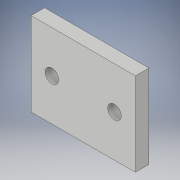
# Autodesk Inventor part: Bed Plate
Saved by Autodesk Inventor 2018 (Build 220112000, 112)
## iProperties
Created: 2017-04-14
Part Number: Bed Plate
Material: Generic
Document SubType Name: Modeling
Designer: Administrator
Density: 1 g/cm^3
Appearance: Default
Author: Administrator
Autodesk Inventor part; units mm, degrees
ref_plane "YZ Plane" through (0, 0, 0) normal (1, 0, 0) x (0, 1, 0)
ref_plane "XZ Plane" through (0, 0, 0) normal (0, 1, 0) x (-1, 0, 0)
ref_plane "XY Plane" through (0, 0, 0) normal (0, 0, 1) x (1, 0, 0)
sketch "Sketch1" plane through (0, 0, 0) normal (0, 0, 1) x (1, 0, 0)
  line L0 (-25, -20) -> (25, -20)
  line L1 (25, -20) -> (25, 20)
  line L2 (25, 20) -> (-25, 20)
  line L3 (-25, 20) -> (-25, -20)
  point P0 (0, 0)
  dimension "d0" = 50
  dimension "d1" = 40
  constraints: 8 end point, 2 parallel, 1 horizontal, 1 perpendicular
  measures "d0" distance of L2.end L1.end
  measures "d1" distance of L1.end L0.end
extrude "Extrusion1" add sketch "Sketch1" along normal blind 6.5
sketch "Sketch2" plane through (0, 0, 6.5) normal (0, 0, 1) x (1, 0, 0)
  circle A0 centre (-15, 0) radius 3.25
  point P0 (0, 0)
  dimension "d4" = 6.5
  constraints: 1 centre point
  measures "d4" diameter of A0
hole "Hole1" at (-15, 0, 6.5) direction (0, 0, -1) diameter 6.5 end through all
sketch "Sketch3" plane through (0, 0, 6.5) normal (0, 0, 1) x (1, 0, 0)
  circle A0 centre (15, 0) radius 3.25
  point P0 (0, 0)
  dimension "d12" = 6.5
  constraints: 1 centre point
  measures "d12" diameter of A0
hole "Hole2" at (15, 0, 6.5) direction (0, 0, -1) diameter 6.5 end through all
body "Solid1"
